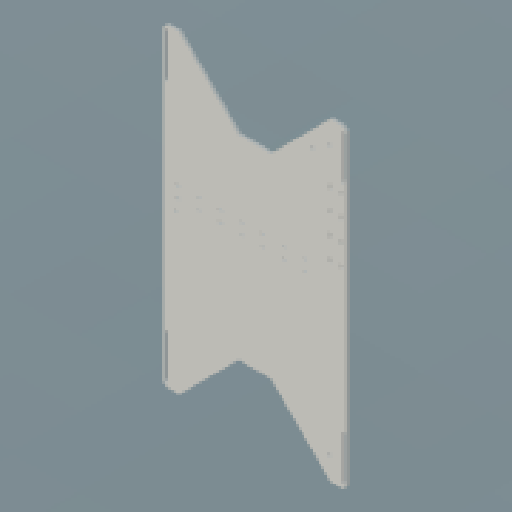
# Autodesk Inventor part: Bed Carrier
Saved by Autodesk Inventor 2023.2 (Build 272271000, 271)
## iProperties
Created: 2023-02-18
Part Number: Bed Carrier
Material: Aluminum 6061
Document SubType Name: Modeling
Designer: remop
Density: 2.7 g/cm^3
Appearance: Aluminum - Flat
Mass: 640.774 g
Surface Area: 1631.54 cm^2
Volume: 237.324 cm^3
Author: remop
Autodesk Inventor part; units mm, degrees
ref_plane "YZ Plane" through (0, 0, 0) normal (1, 0, 0) x (0, 1, 0)
ref_plane "XZ Plane" through (0, 0, 0) normal (0, 1, 0) x (-1, 0, 0)
ref_plane "XY Plane" through (0, 0, 0) normal (0, 0, 1) x (1, 0, 0)
sketch "Sketch1" plane through (0, 0, 0) normal (0, 0, 1) x (1, 0, 0)
  arc A0 (-138.7058, 176.7669) -> (-140.7058, 174.7669) centre (-138.7058, 174.7669) ccw projected
  line L0 (-138.7058, 176.7669) -> (73.2942, 176.7669) projected
  arc A1 (75.2942, 174.7669) -> (73.2942, 176.7669) centre (73.2942, 174.7669) ccw projected
  line L1 (75.2942, 174.7669) -> (75.2942, -135.2331) projected
  arc A2 (73.2942, -137.2331) -> (75.2942, -135.2331) centre (73.2942, -135.2331) ccw projected
  line L2 (73.2942, -137.2331) -> (-138.7058, -137.2331) projected
  arc A3 (-140.7058, -135.2331) -> (-138.7058, -137.2331) centre (-138.7058, -135.2331) ccw projected
  line L3 (-140.7058, -135.2331) -> (-140.7058, 174.7669) projected
  arc A4 (-135.5477, 174.3853) -> (-138.8639, 172.1485) centre (-137.2058, 173.2669) ccw projected
  line L4 (-138.8639, 172.1485) -> (-134.67, 165.9308) projected
  arc A5 (-134.67, 165.9308) -> (-131.3538, 168.1675) centre (-133.0119, 167.0491) ccw projected
  line L5 (-131.3538, 168.1675) -> (-135.5477, 174.3853) projected
  line L6 (-135.5477, -134.8515) -> (-131.3538, -128.6337) projected
  arc A6 (-131.3538, -128.6337) -> (-134.67, -126.3969) centre (-133.0119, -127.5153) ccw projected
  line L7 (-134.67, -126.3969) -> (-138.8639, -132.6147) projected
  arc A7 (-138.8639, -132.6147) -> (-135.5477, -134.8515) centre (-137.2058, -133.7331) ccw projected
  arc A8 (69.2583, -126.3969) -> (65.9422, -128.6337) centre (67.6002, -127.5153) ccw projected
  line L8 (65.9422, -128.6337) -> (70.1361, -134.8515) projected
  arc A9 (70.1361, -134.8515) -> (73.4523, -132.6147) centre (71.7942, -133.7331) ccw projected
  line L9 (73.4523, -132.6147) -> (69.2583, -126.3969) projected
  line L10 (70.1361, 174.3853) -> (65.9422, 168.1675) projected
  arc A10 (65.9422, 168.1675) -> (69.2583, 165.9308) centre (67.6002, 167.0491) ccw projected
  line L11 (69.2583, 165.9308) -> (73.4523, 172.1485) projected
  arc A11 (73.4523, 172.1485) -> (70.1361, 174.3853) centre (71.7942, 173.2669) ccw projected
  line L12 (-140.7058, 174.7669) -> (-140.7058, 204.7669)
  line L13 (-140.7058, 204.7669) -> (75.2942, 204.7669)
  line L14 (75.2942, 204.7669) -> (75.2942, 174.7669)
  line L15 (75.2942, -135.2331) -> (75.2942, -165.2331)
  line L16 (75.2942, -165.2331) -> (-140.7058, -165.2331)
  line L17 (-140.7058, -135.2331) -> (-140.7058, -165.2331)
  line L18 (71.7942, 148.2669) -> (71.7942, 198.2669) construction
  line L19 (73.5442, 148.2669) -> (73.5442, 198.2669)
  line L20 (70.0442, 198.2669) -> (70.0442, 148.2669)
  arc A12 (70.0442, 148.2669) -> (73.5442, 148.2669) centre (71.7942, 148.2669) ccw
  arc A13 (73.5442, 198.2669) -> (70.0442, 198.2669) centre (71.7942, 198.2669) ccw
  line L21 (-137.2058, 148.2669) -> (-137.2058, 198.2669) construction
  line L22 (-138.9558, 148.2669) -> (-138.9558, 198.2669)
  line L23 (-135.4558, 198.2669) -> (-135.4558, 148.2669)
  arc A14 (-138.9558, 148.2669) -> (-135.4558, 148.2669) centre (-137.2058, 148.2669) ccw
  arc A15 (-135.4558, 198.2669) -> (-138.9558, 198.2669) centre (-137.2058, 198.2669) ccw
  line L24 (-137.2058, -158.7331) -> (-137.2058, -108.7331) construction
  line L25 (-135.4558, -158.7331) -> (-135.4558, -108.7331)
  line L26 (-138.9558, -108.7331) -> (-138.9558, -158.7331)
  arc A16 (-138.9558, -158.7331) -> (-135.4558, -158.7331) centre (-137.2058, -158.7331) ccw
  arc A17 (-135.4558, -108.7331) -> (-138.9558, -108.7331) centre (-137.2058, -108.7331) ccw
  line L27 (71.7942, -108.7331) -> (71.7942, -158.7331) construction
  line L28 (73.5442, -108.7331) -> (73.5442, -158.7331)
  line L29 (70.0442, -158.7331) -> (70.0442, -108.7331)
  arc A18 (73.5442, -108.7331) -> (70.0442, -108.7331) centre (71.7942, -108.7331) ccw
  arc A19 (70.0442, -158.7331) -> (73.5442, -158.7331) centre (71.7942, -158.7331) ccw
  point P0 (0, 0)
  point P1 (70.0442, -134.7152)
  point P2 (70.0442, -127.562)
  dimension "d13" = 30
  dimension "d14" = 3.5
  dimension "d15" = 50
  constraints: 44 end point, 16 point on circle, 16 tangent, 8 centre point, 6 parallel, 5 equal length, 4 midpoint, 4 vertical, 3 equal radius, 2 perpendicular, 2 point on line
  measures "d13" distance of L3.start L16.end
  measures "d14" distance between parallel lines of L19 L20
  measures "d15" distance of L20.start L20.end
extrude "Extrusion1" add sketch "Sketch1" along normal blind 3 contours L22 A4 A14 L23 L4 A5 L5 L0 L20 L10 A10 L11 A12 L19 A11 A1 L1 A2 L28 A9 A18 L29 L9 A8 L8 L2 L25 L6 A6 L7 A17 L26 A7 A3 L3 A0 | A0 L12 L13 L14 A1 L19 A13 L20 L0 L23 A15 L22 | L22 A4 | L5 A5 L4 L23 | A3 L26 A16 L25 L2 L29 A19 L28 A2 L15 L16 L17 | L20 L11 A10 L10 | A7 L26 | A11 L19 | L25 L7 A6 L6 | L8 A8 L9 L29 | L28 A9
sketch "Sketch2" plane through (0, 0, 0) normal (0, 0, -1) x (-1, 0, 0)
  line L0 (-70.0442, -158.7331) -> (-70.0442, -108.7331) projected
  arc A0 (-70.0442, -108.7331) -> (-73.5442, -108.7331) centre (-71.7942, -108.7331) ccw projected
  line L1 (-73.5442, -108.7331) -> (-73.5442, -158.7331) projected
  arc A1 (-73.5442, -158.7331) -> (-70.0442, -158.7331) centre (-71.7942, -158.7331) ccw projected
  line L2 (-75.2942, 204.7669) -> (140.7058, 204.7669) projected
  line L3 (-75.2942, -165.2331) -> (-75.2942, 204.7669) projected
  line L4 (140.7058, -165.2331) -> (-75.2942, -165.2331) projected
  line L5 (140.7058, 204.7669) -> (140.7058, -165.2331) projected
  line L6 (-73.5442, 198.2669) -> (-73.5442, 148.2669) projected
  arc A2 (-70.0442, 198.2669) -> (-73.5442, 198.2669) centre (-71.7942, 198.2669) ccw projected
  line L7 (-70.0442, 148.2669) -> (-70.0442, 198.2669) projected
  arc A3 (-73.5442, 148.2669) -> (-70.0442, 148.2669) centre (-71.7942, 148.2669) ccw projected
  line L8 (135.4558, 198.2669) -> (135.4558, 148.2669) projected
  arc A4 (138.9558, 198.2669) -> (135.4558, 198.2669) centre (137.2058, 198.2669) ccw projected
  line L9 (138.9558, 148.2669) -> (138.9558, 198.2669) projected
  arc A5 (135.4558, 148.2669) -> (138.9558, 148.2669) centre (137.2058, 148.2669) ccw projected
  line L10 (138.9558, -158.7331) -> (138.9558, -108.7331) projected
  arc A6 (135.4558, -158.7331) -> (138.9558, -158.7331) centre (137.2058, -158.7331) ccw projected
  line L11 (135.4558, -108.7331) -> (135.4558, -158.7331) projected
  arc A7 (138.9558, -108.7331) -> (135.4558, -108.7331) centre (137.2058, -108.7331) ccw projected
  line L12 (-70.0442, -158.7331) -> (-70.0442, -108.7331) projected
  arc A8 (-73.5442, -158.7331) -> (-70.0442, -158.7331) centre (-71.7942, -158.7331) ccw projected
  line L13 (-73.5442, -108.7331) -> (-73.5442, -158.7331) projected
  arc A9 (-70.0442, -108.7331) -> (-73.5442, -108.7331) centre (-71.7942, -108.7331) ccw projected
  line L14 (140.7058, 204.7669) -> (140.7058, -165.2331) projected
  point P0 (0, 0)
  point P1 (-55.2942, -138.2331)
  point P2 (-55.2942, 177.7669)
  point P3 (125.7058, 19.7669)
  point P4 (140.7058, 19.7669)
  point P5 (140.7058, 19.7669)
  dimension "d17" = 15
  dimension "d18" = 27
  dimension "d19" = 20
  dimension "d20" = 27
  constraints: 2 midpoint, 1 horizontal alignment, 1 vertical alignment
  measures "d17" distance of point (125.706, 19.767) point (140.706, 19.767)
  measures "d18" distance from line of L2 point (-55.294, 177.767)
  measures "d19" distance from line of L3 point (-55.294, 177.767)
  measures "d20" distance from line of L4 point (-55.294, -138.233)
hole "Hole1" at (55.2942, -138.2331, 0) at (55.2942, 177.7669, 0) at (-125.7058, 19.7669, 0) direction (0, 0, 1) diameter 4.2 end through all
chamfer "Chamfer1" distance 4 angle 45 4 edges at (75.2942, 204.7669, 1.5) (75.2942, -165.2331, 1.5) (-140.7058, -165.2331, 1.5) (-140.7058, 204.7669, 1.5)
sketch "Sketch3" plane through (0, 0, 0) normal (0, 0, -1) x (-1, 0, 0)
  line L0 (136.7058, 204.7669) -> (140.7058, 200.7669) projected
  line L1 (-71.2942, 204.7669) -> (136.7058, 204.7669) projected
  line L2 (-75.2942, 200.7669) -> (-71.2942, 204.7669) projected
  line L3 (-75.2942, -161.2331) -> (-75.2942, 200.7669) projected
  line L4 (-71.2942, -165.2331) -> (-75.2942, -161.2331) projected
  line L5 (136.7058, -165.2331) -> (-71.2942, -165.2331) projected
  line L6 (140.7058, -161.2331) -> (136.7058, -165.2331) projected
  line L7 (140.7058, 200.7669) -> (140.7058, -161.2331) projected
  circle A0 centre (-55.2942, 177.7669) radius 2.1 projected
  circle A1 centre (-55.2942, -138.2331) radius 2.1 projected
  circle A2 centre (125.7058, 19.7669) radius 2.1 projected
  line L8 (-73.5442, 198.2669) -> (-73.5442, 148.2669) projected
  arc A3 (-70.0442, 198.2669) -> (-73.5442, 198.2669) centre (-71.7942, 198.2669) ccw projected
  line L9 (-70.0442, 148.2669) -> (-70.0442, 198.2669) projected
  arc A4 (-73.5442, 148.2669) -> (-70.0442, 148.2669) centre (-71.7942, 148.2669) ccw projected
  line L10 (135.4558, 198.2669) -> (135.4558, 148.2669) projected
  arc A5 (138.9558, 198.2669) -> (135.4558, 198.2669) centre (137.2058, 198.2669) ccw projected
  line L11 (138.9558, 148.2669) -> (138.9558, 198.2669) projected
  arc A6 (135.4558, 148.2669) -> (138.9558, 148.2669) centre (137.2058, 148.2669) ccw projected
  line L12 (138.9558, -158.7331) -> (138.9558, -108.7331) projected
  arc A7 (135.4558, -158.7331) -> (138.9558, -158.7331) centre (137.2058, -158.7331) ccw projected
  line L13 (135.4558, -108.7331) -> (135.4558, -158.7331) projected
  arc A8 (138.9558, -108.7331) -> (135.4558, -108.7331) centre (137.2058, -108.7331) ccw projected
  line L14 (-70.0442, -158.7331) -> (-70.0442, -108.7331) projected
  arc A9 (-73.5442, -158.7331) -> (-70.0442, -158.7331) centre (-71.7942, -158.7331) ccw projected
  line L15 (-73.5442, -108.7331) -> (-73.5442, -158.7331) projected
  arc A10 (-70.0442, -108.7331) -> (-73.5442, -108.7331) centre (-71.7942, -108.7331) ccw projected
  line L16 (-57.2942, 133.2669) -> (-55.2942, 133.2669)
  line L17 (-55.2942, 133.2669) -> (-55.2942, 138.2669)
  line L18 (-55.2942, 138.2669) -> (-57.2942, 138.2669)
  line L19 (-57.2942, 138.2669) -> (-57.2942, 133.2669)
  line L20 (-70.2942, 133.2669) -> (-68.2942, 133.2669)
  line L21 (-68.2942, 133.2669) -> (-68.2942, 138.2669)
  line L22 (-68.2942, 138.2669) -> (-70.2942, 138.2669)
  line L23 (-70.2942, 138.2669) -> (-70.2942, 133.2669)
  line L24 (-68.2942, 108.2669) -> (-68.2942, 113.2669)
  line L25 (-70.2942, 108.2669) -> (-68.2942, 108.2669)
  line L26 (-70.2942, 113.2669) -> (-70.2942, 108.2669)
  line L27 (-68.2942, 113.2669) -> (-70.2942, 113.2669)
  line L28 (-57.2942, 113.2669) -> (-57.2942, 108.2669)
  line L29 (-55.2942, 113.2669) -> (-57.2942, 113.2669)
  line L30 (-57.2942, 108.2669) -> (-55.2942, 108.2669)
  line L31 (-55.2942, 108.2669) -> (-55.2942, 113.2669)
  line L32 (-68.2942, 83.2669) -> (-68.2942, 88.2669)
  line L33 (-70.2942, 83.2669) -> (-68.2942, 83.2669)
  line L34 (-70.2942, 88.2669) -> (-70.2942, 83.2669)
  line L35 (-68.2942, 88.2669) -> (-70.2942, 88.2669)
  line L36 (-57.2942, 88.2669) -> (-57.2942, 83.2669)
  line L37 (-55.2942, 88.2669) -> (-57.2942, 88.2669)
  line L38 (-57.2942, 83.2669) -> (-55.2942, 83.2669)
  line L39 (-55.2942, 83.2669) -> (-55.2942, 88.2669)
  line L40 (-68.2942, 58.2669) -> (-68.2942, 63.2669)
  line L41 (-70.2942, 58.2669) -> (-68.2942, 58.2669)
  line L42 (-70.2942, 63.2669) -> (-70.2942, 58.2669)
  line L43 (-68.2942, 63.2669) -> (-70.2942, 63.2669)
  line L44 (-57.2942, 63.2669) -> (-57.2942, 58.2669)
  line L45 (-55.2942, 63.2669) -> (-57.2942, 63.2669)
  line L46 (-57.2942, 58.2669) -> (-55.2942, 58.2669)
  line L47 (-55.2942, 58.2669) -> (-55.2942, 63.2669)
  line L48 (-68.2942, 33.2669) -> (-68.2942, 38.2669)
  line L49 (-70.2942, 33.2669) -> (-68.2942, 33.2669)
  line L50 (-70.2942, 38.2669) -> (-70.2942, 33.2669)
  line L51 (-68.2942, 38.2669) -> (-70.2942, 38.2669)
  line L52 (-57.2942, 38.2669) -> (-57.2942, 33.2669)
  line L53 (-55.2942, 38.2669) -> (-57.2942, 38.2669)
  line L54 (-57.2942, 33.2669) -> (-55.2942, 33.2669)
  line L55 (-55.2942, 33.2669) -> (-55.2942, 38.2669)
  line L56 (125.7058, 33.2669) -> (120.7058, 33.2669)
  line L57 (120.7058, 33.2669) -> (120.7058, 35.2669)
  line L58 (120.7058, 35.2669) -> (125.7058, 35.2669)
  line L59 (125.7058, 35.2669) -> (125.7058, 33.2669)
  line L60 (125.7058, 46.2669) -> (120.7058, 46.2669)
  line L61 (120.7058, 46.2669) -> (120.7058, 48.2669)
  line L62 (120.7058, 48.2669) -> (125.7058, 48.2669)
  line L63 (125.7058, 48.2669) -> (125.7058, 46.2669)
  line L64 (95.7058, 48.2669) -> (100.7058, 48.2669)
  line L65 (100.7058, 48.2669) -> (100.7058, 46.2669)
  line L66 (95.7058, 46.2669) -> (95.7058, 48.2669)
  line L67 (100.7058, 46.2669) -> (95.7058, 46.2669)
  line L68 (95.7058, 35.2669) -> (100.7058, 35.2669)
  line L69 (100.7058, 35.2669) -> (100.7058, 33.2669)
  line L70 (95.7058, 33.2669) -> (95.7058, 35.2669)
  line L71 (100.7058, 33.2669) -> (95.7058, 33.2669)
  line L72 (70.7058, 48.2669) -> (75.7058, 48.2669)
  line L73 (75.7058, 48.2669) -> (75.7058, 46.2669)
  line L74 (70.7058, 46.2669) -> (70.7058, 48.2669)
  line L75 (75.7058, 46.2669) -> (70.7058, 46.2669)
  line L76 (70.7058, 35.2669) -> (75.7058, 35.2669)
  line L77 (75.7058, 35.2669) -> (75.7058, 33.2669)
  line L78 (70.7058, 33.2669) -> (70.7058, 35.2669)
  line L79 (75.7058, 33.2669) -> (70.7058, 33.2669)
  line L80 (45.7058, 48.2669) -> (50.7058, 48.2669)
  line L81 (50.7058, 48.2669) -> (50.7058, 46.2669)
  line L82 (45.7058, 46.2669) -> (45.7058, 48.2669)
  line L83 (50.7058, 46.2669) -> (45.7058, 46.2669)
  line L84 (45.7058, 35.2669) -> (50.7058, 35.2669)
  line L85 (50.7058, 35.2669) -> (50.7058, 33.2669)
  line L86 (45.7058, 33.2669) -> (45.7058, 35.2669)
  line L87 (50.7058, 33.2669) -> (45.7058, 33.2669)
  line L88 (20.7058, 48.2669) -> (25.7058, 48.2669)
  line L89 (25.7058, 48.2669) -> (25.7058, 46.2669)
  line L90 (20.7058, 46.2669) -> (20.7058, 48.2669)
  line L91 (25.7058, 46.2669) -> (20.7058, 46.2669)
  line L92 (20.7058, 35.2669) -> (25.7058, 35.2669)
  line L93 (25.7058, 35.2669) -> (25.7058, 33.2669)
  line L94 (20.7058, 33.2669) -> (20.7058, 35.2669)
  line L95 (25.7058, 33.2669) -> (20.7058, 33.2669)
  line L96 (-4.2942, 48.2669) -> (0.7058, 48.2669)
  line L97 (0.7058, 48.2669) -> (0.7058, 46.2669)
  line L98 (-4.2942, 46.2669) -> (-4.2942, 48.2669)
  line L99 (0.7058, 46.2669) -> (-4.2942, 46.2669)
  line L100 (-4.2942, 35.2669) -> (0.7058, 35.2669)
  line L101 (0.7058, 35.2669) -> (0.7058, 33.2669)
  line L102 (-4.2942, 33.2669) -> (-4.2942, 35.2669)
  line L103 (0.7058, 33.2669) -> (-4.2942, 33.2669)
  line L104 (-29.2942, 48.2669) -> (-24.2942, 48.2669)
  line L105 (-24.2942, 48.2669) -> (-24.2942, 46.2669)
  line L106 (-29.2942, 46.2669) -> (-29.2942, 48.2669)
  line L107 (-24.2942, 46.2669) -> (-29.2942, 46.2669)
  line L108 (-29.2942, 35.2669) -> (-24.2942, 35.2669)
  line L109 (-24.2942, 35.2669) -> (-24.2942, 33.2669)
  line L110 (-29.2942, 33.2669) -> (-29.2942, 35.2669)
  line L111 (-24.2942, 33.2669) -> (-29.2942, 33.2669)
  line L112 (-71.2942, 204.7669) -> (136.7058, 204.7669) projected
  line L113 (121.7058, 204.7669) -> (51.7058, 134.7669)
  line L114 (51.7058, 134.7669) -> (13.7058, 134.7669)
  line L115 (13.7058, 134.7669) -> (-56.2942, 204.7669)
  line L116 (136.7058, 204.7669) -> (140.7058, 200.7669) projected
  line L117 (-75.2942, 200.7669) -> (-71.2942, 204.7669) projected
  line L118 (136.7058, -165.2331) -> (-71.2942, -165.2331) projected
  line L119 (121.7058, -165.2331) -> (51.7058, -95.2331)
  line L120 (51.7058, -95.2331) -> (13.7058, -95.2331)
  line L121 (13.7058, -95.2331) -> (-56.2942, -165.2331)
  line L122 (140.7058, -161.2331) -> (136.7058, -165.2331) projected
  line L123 (-71.2942, -165.2331) -> (-75.2942, -161.2331) projected
  circle A11 centre (-35.2942, 164.7669) radius 2.25
  point P0 (0, 0)
  point P1 (-55.2942, 135.7669)
  point P2 (-70.2942, 135.7669)
  point P3 (-56.2942, 133.2669)
  point P4 (-69.2942, 133.2669)
  point P5 (-69.2942, 108.2669)
  point P6 (-70.2942, 110.7669)
  point P7 (-56.2942, 108.2669)
  point P8 (-55.2942, 110.7669)
  point P9 (-69.2942, 83.2669)
  point P10 (-70.2942, 85.7669)
  point P11 (-56.2942, 83.2669)
  point P12 (-55.2942, 85.7669)
  point P13 (-69.2942, 58.2669)
  point P14 (-70.2942, 60.7669)
  point P15 (-56.2942, 58.2669)
  point P16 (-55.2942, 60.7669)
  point P17 (-69.2942, 33.2669)
  point P18 (-70.2942, 35.7669)
  point P19 (-56.2942, 33.2669)
  point P20 (-55.2942, 35.7669)
  point P21 (-69.2942, 138.2669)
  dimension "d34" = 25
  dimension "d39" = 5
  dimension "d40" = 2
  dimension "d41" = 10
  dimension "d42" = 5
  dimension "d43" = 15
  dimension "d44" = 15
  dimension "d45" = 15
  dimension "d48" = 25
  dimension "d56" = 15
  dimension "d57" = 15
  dimension "d58" = 70
  dimension "d59" = 4.5
  dimension "d60" = 40
  dimension "d61" = 40
  constraints: 204 end point, 18 point on line, 10 parallel, 9 perpendicular, 5 equal length, 5 horizontal, 5 midpoint, 3 vertical alignment, 2 horizontal alignment, 1 centre point, 1 vertical, 176 other
  measures "d34" distance of L20.end L24.start
  measures "d39" distance between parallel lines of L3 L23
  measures "d40" distance of L21.end L22.end
  measures "d41" vertical distance of A4.centre point (-69.294, 138.267)
  measures "d42" distance of L20.end L21.end
  measures "d43" distance between parallel lines of L62 L56
  measures "d44" distance between parallel lines of L23 L17
  measures "d45" distance between parallel lines of L7 L63
  measures "d48" distance of L62.end L64.end
  measures "d56" distance of L1.start L115.end
  measures "d57" distance of L0.start L113.start
  measures "d58" distance between parallel lines of L1 L114
  measures "d59" diameter of A11
  measures "d60" distance from line of L3 A11.centre
  measures "d61" distance from line of L1 A11.centre
extrude "Extrusion2" cut sketch "Sketch3" against normal through all contours L113 L114 L115 L1 | L5 L121 L120 L119 | L19 L18 L17 L16 | L23 L22 L21 L20 | L25 L26 L27 L24 | L29 L31 L30 L28 | L33 L34 L35 L32 | L37 L39 L38 L36 | L41 L42 L43 L40 | L45 L47 L46 L44 | L56 L57 L58 L59 | L60 L61 L62 L63 | L64 L65 L67 L66 | L68 L69 L71 L70 | L72 L73 L75 L74 | L76 L77 L79 L78 | L80 L81 L83 L82 | L84 L85 L87 L86 | L88 L89 L91 L90 | L92 L93 L95 L94 | L96 L97 L99 L98 | L100 L101 L103 L102 | L104 L105 L107 L106 | L108 L109 L111 L110 | A11
equation "\"d20\" = d18"
equation "\"d44\" = d43"
equation "\"d57\" = d56"
equation "\"d61\" = d60"
body "Solid1"
